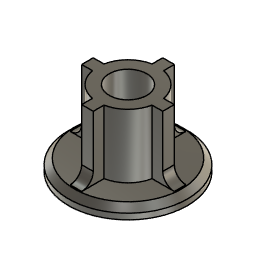
screw_guide_piece (Autodesk Fusion 360 design; units mm, degrees)
Autodesk Fusion 360 part; units mm, degrees
note: some values were not read from the file. Set by a fixed rule: which sketch regions a step uses.
sketch "Sketch1" plane through (0, 0, 0) normal (0, 0, 1) x (1, 0, 0)
  circle A0 centre (0, 0) radius 3.25
  circle A1 centre (0, 0) radius 9.25
  dimension "d1" = 6.5
  dimension "d2" = 6
  constraint coincident A0.centre A1.centre
  measures "d1" diameter of A0
extrude "Extrude1" add sketch "Sketch1" along normal blind 2
sketch "Sketch2" plane through (0, 0, 2) normal (0, 0, 1) x (-1, 0, 0)
  circle A0 centre (0, 0) radius 3.25
  circle A1 centre (0, 0) radius 9.25
  circle A2 centre (0, 0) radius 5.25
  line L0 (-7, -1) -> (7, -1)
  line L1 (7, -1) -> (7, 1)
  line L2 (7, 1) -> (-7, 1)
  line L3 (-7, 1) -> (-7, -1)
  line L4 (-7, -1) -> (7, 1) construction
  line L5 (7, -1) -> (-7, 1) construction
  line L6 (-1, -7) -> (1, -7)
  line L7 (1, -7) -> (1, 7)
  line L8 (1, 7) -> (-1, 7)
  line L9 (-1, 7) -> (-1, -7)
  line L10 (-1, -7) -> (1, 7) construction
  line L11 (1, -7) -> (-1, 7) construction
  dimension "d5" = 2
  dimension "d6" = 14
  dimension "d7" = 2
  dimension "d8" = 2
  dimension "d9" = 14
  constraint horizontal L0
  constraint perpendicular L0 L1
  constraint parallel L0 L2
  constraint parallel L1 L3
  constraint coincident L4 A0.centre
  constraint coincident L5 A0.centre
  constraint coincident A0.centre A1.centre
  constraint horizontal L6
  constraint perpendicular L6 L7
  constraint parallel L6 L8
  constraint parallel L7 L9
  constraint coincident L10 A0.centre
  constraint coincident L11 A0.centre
  measures "d6" distance of L1.end L2.end
  measures "d7" distance of L0.end L1.end
  measures "d8" distance of L7.end L8.end
  measures "d9" distance of L6.end L7.end
extrude "Extrude2" add sketch "Sketch2" along normal blind 11 contours A0 A2 L0 L2 | A0 A2 L2 L7 | A0 A2 L0 L7 | A0 A2 L7 L9 | A2 L0 L1 L2 | A0 A2 L7 L9 | A0 A2 L2 L9 | A2 L7 L8 L9 | A0 A2 L0 L9 | A2 L6 L7 L9 | A0 A2 L0 L2 | A2 L0 L2 L3
chamfer "Chamfer1" distance 1 angle 45 1 edges at (-8.624, -3.3449, 2)
move_face "OffsetFaces1" offset 1 1 faces at (9.2385, -0.4611, 0.6667)
fillet "Fillet1" radius 2 4 edges at (0, -7, 2) (-7, 0, 2) (0, 7, 2) (7, 0, 2)
named bodies: "peca_sanita"
